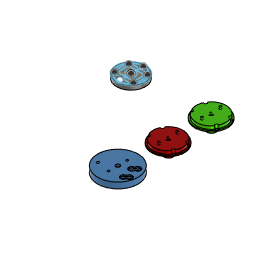
2023_05_26_IMacG4TopPart1 Fail v1 (Autodesk Fusion 360 design; units mm, degrees)
Autodesk Fusion 360 part; units mm, degrees
sketch "Screw Dim" plane through (0, 0, 0) normal (0, 0, 1) x (1, 0, 0)
  circle A0 centre (0, 0) radius 3.5
  circle A1 centre (0, 0) radius 1.755
  dimension "d1" = 7
  dimension "d2" = 3.51
  constraint coincident A0.centre A1.centre
  constraint concentric A0 A1
  measures "d1" diameter of A0
  measures "d2" diameter of A1
extrude "Extrude1" add sketch "Screw Dim" along normal blind 5 contours A0 | A1 makes body 1
extrude "Extrude2" cut sketch "Screw Dim" along normal blind 3.8 bodies 1
move_body "Move1" bodies 1 to x (1, 0, 0) y (0, 1, 0) z (0, 0, 1) at (0, 50, 0)
sketch "Sketch2" plane through (0, 0, 0) normal (0, 0, 1) x (1, 0, 0)
  line L0 (0, 0) -> (22.6, 0) construction
  line L1 (-10.9513, 2.215) -> (-10.9513, 17.585) construction
  line L2 (-10.9513, 9.9) -> (-10.9513, 22.015) construction
  line L3 (-10.9513, 9.9) -> (-10.9513, -2.215) construction
  line L4 (11.3, 0) -> (26.3, 0) construction
  line L5 (11.3, 0) -> (-3.7, 0) construction
  line L6 (-10.9513, 2.215) -> (-10.9513, -2.215) construction
  line L7 (-10.9513, 22.015) -> (-10.9513, 17.585) construction
  line L8 (26.3, 0) -> (22.6, 0) construction
  line L9 (-10.9513, 19.8) -> (24.45, 19.8) construction
  line L10 (24.45, 19.8) -> (24.45, 0) construction
  circle A0 centre (-10.9513, 19.8) radius 2.215
  circle A1 centre (24.45, 19.8) radius 2.215
  circle A2 centre (24.45, 0) radius 2.215
  circle A3 centre (-10.9513, 0) radius 2.215
  line L11 (-10.9513, 19.8) -> (24.45, 0) construction
  line L12 (24.45, 19.8) -> (-10.9513, 0) construction
  line L13 (6.7494, 9.9) -> (6.7494, 21.3) construction
  line L14 (6.7494, 9.9) -> (6.7494, 24.3) construction
  line L15 (6.7494, 21.3) -> (6.7494, 24.3) construction
  line L16 (6.7494, 9.9) -> (6.7494, -3.45) construction
  circle A4 centre (6.7494, 9.9) radius 2.875
  circle A5 centre (6.7494, 9.9) radius 11.35
  circle A6 centre (6.7494, 9.9) radius 20.6
  circle A7 centre (6.7494, 9.9) radius 22.6
  line L17 (0, 0) -> (-3.7, 0)
  circle A8 centre (6.7494, 22.8) radius 1.5
  circle A9 centre (6.7494, -3) radius 1.5
  line L18 (-10.9513, 22.015) -> (-10.9513, -2.215)
  point P0 (-10.9513, 0)
  point P1 (-10.9513, 0)
  point P2 (-1.85, 0)
  dimension "d10" = 22.6
  dimension "d11" = 15.37
  dimension "d12" = 12.115
  dimension "d13" = 12.115
  dimension "d14" = 15
  dimension "d15" = 14.4
  dimension "d16" = 11.4
  dimension "d18" = 5.75
  dimension "d19" = 41.2
  dimension "d20" = 45.2
  dimension "d56" = 360
  dimension "d66" = 24.23
  constraint coincident L0.start L17.start
  constraint horizontal L0
  constraint vertical L1
  constraint coincident L1 L2.start
  constraint parallel L1 L2
  constraint parallel L1 L3
  constraint midpoint L1 L2.start
  constraint midpoint L0 L4.start
  constraint parallel L0 L4
  constraint parallel L0 L5
  constraint equal L4 L5
  constraint coincident L5 P1
  constraint midpoint L6 P1
  constraint coincident P1 P0
  constraint midpoint L7 L9.start
  constraint perpendicular L7 L9
  constraint midpoint L8 L10.end
  constraint perpendicular L8 L10
  constraint coincident L9.start A0.centre
  constraint coincident L1.end A0
  constraint coincident L9.end L10.start
  constraint coincident L10.end A2.centre
  constraint equal A0 A1
  constraint equal A0 A3
  constraint equal A0 A2
  constraint midpoint L11 L13.start
  constraint perpendicular L9 L13
  constraint parallel L13 L14
  constraint parallel L14 L16
  constraint coincident L13.start L14.start
  constraint concentric A4 A5
  constraint concentric A4 A6
  constraint concentric A5 A7
  constraint midpoint L17 P2
  constraint coincident L14.end A8
  constraint coincident L13.end A8
  measures "d10" distance of L0.start L0.end
  measures "d11" distance of L1.start L1.end
  measures "d12" distance of L2.start L2.end
  measures "d13" distance of L2.start L3.end
  measures "d14" distance of L4.start L4.end
  measures "d15" distance of L13.start L14.end
  measures "d16" distance of L13.start L13.end
  measures "d18" diameter of A4
  measures "d19" diameter of A6
  measures "d20" diameter of A7
  measures "d66" distance of L2.end L3.end
extrude "Extrude3" add sketch "Sketch2" against normal blind 5.75 separate body contours A0 A6 L18 | A0 A1 A2 A3 A6 L18 | A0 A6 L18 | A0 A3 A6 L18 | A0 A6 L18 | A0 A6 L18 | A1 A6 | A1 A6 | A3 A6 L18 | A3 A6 L18 | A3 A6 L18 | A3 A6 L18 | A2 A6 | A2 A6 | A4 | A5 | A7 | A8 | A9 makes body 2
extrude "Extrude4" cut sketch "Sketch2" against normal blind 4.15 contours A0 A6 L18 | A0 A6 L18 | A1 A6 | A3 A6 L18 | A3 A6 L18 | A2 A6 | A7 picked at (-10.6589, 21.4307) picked at (-11.7417, 20.3274) picked at (25.2501, 20.2971) picked at (-11.7417, -0.5274) picked at (-10.6589, -1.6307) picked at (25.2501, -0.4971) bodies 2
extrude "Extrude5" cut sketch "Sketch2" against normal blind 5.2 contours A0 A6 L18 | A0 A6 L18 | A0 A6 L18 | A0 A6 L18 | A1 A6 | A1 A6 | A3 A6 L18 | A3 A6 L18 | A3 A6 L18 | A3 A6 L18 | A2 A6 | A2 A6 bodies 2
extrude "Extrude6" add sketch "Sketch2" along normal blind 2.5 contours A8 | A9 bodies 2
extrude "Extrude7" cut sketch "Sketch2" against normal blind 28 contours A4 bodies 2
sketch "Sketch10" plane through (0, 0, 0) normal (0, 0, 1) x (1, 0, 0)
  line L0 (-82.5, 14.73) -> (-112.5, 14.73)
  line L1 (-112.5, 14.73) -> (-112.5, -9.5)
  line L2 (-112.5, -9.5) -> (-82.5, -9.5)
  line L3 (-82.5, -9.5) -> (-82.5, 14.73)
  line L4 (-82.5, 14.73) -> (-112.5, -9.5) construction
  line L5 (-112.5, 14.73) -> (-82.5, -9.5) construction
  line L6 (-86.2, 10.3) -> (-108.8, 10.3)
  line L7 (-108.8, 10.3) -> (-108.8, -5.07)
  line L8 (-108.8, -5.07) -> (-86.2, -5.07)
  line L9 (-86.2, -5.07) -> (-86.2, 10.3)
  line L10 (-86.2, 10.3) -> (-108.8, -5.07) construction
  line L11 (-108.8, 10.3) -> (-86.2, -5.07) construction
  line L12 (-97.5, 2.615) -> (-97.5, 16.515)
  line L13 (-97.5, 2.615) -> (-97.5, 19.615)
  line L14 (-108.8, -5.07) -> (-112.5, -5.07) construction
  line L15 (-108.8, -5.07) -> (-108.8, -9.5) construction
  line L16 (-97.5, 19.615) -> (-97.5, -14.385)
  circle A0 centre (-97.5, 18.065) radius 1.55
  circle A1 centre (-97.5, -12.835) radius 1.55
  line L17 (-108.8, 10.3) -> (-112.5, 14.73) construction
  line L18 (-86.2, 10.3) -> (-82.5, 14.73) construction
  line L19 (-86.2, -5.07) -> (-82.5, -9.5) construction
  line L20 (-112.5, -9.5) -> (-108.8, -5.07) construction
  circle A2 centre (-110.65, 12.515) radius 1.7
  circle A3 centre (-84.35, 12.515) radius 1.7
  circle A4 centre (-84.35, -7.285) radius 1.7
  circle A5 centre (-110.65, -7.285) radius 1.7
  point P0 (-97.5, 2.615)
  point P1 (-97.5, 2.615)
  point P2 (-97.5, 19.615)
  dimension "d69" = 30
  dimension "d70" = 24.23
  dimension "d71" = 22.6
  dimension "d72" = 15.37
  dimension "d73" = 13.9
  dimension "d74" = 17
  dimension "d89" = 360
  dimension "d90" = 3.4
  constraint horizontal L0
  constraint perpendicular L0 L1
  constraint parallel L0 L2
  constraint parallel L1 L3
  constraint coincident L4 P1
  constraint coincident L5 P1
  constraint horizontal L6
  constraint perpendicular L6 L7
  constraint parallel L6 L8
  constraint parallel L7 L9
  constraint coincident L10 P1
  constraint coincident L11 P1
  constraint coincident P1 P0
  constraint perpendicular L0 L12
  constraint perpendicular L0 L13
  constraint coincident L1 L14.end
  constraint perpendicular L1 L14
  constraint coincident L2 L15.end
  constraint perpendicular L2 L15
  constraint perpendicular L2 L16
  constraint coincident P2 L13.end
  constraint coincident P2 A0
  constraint coincident L12.end A0
  constraint midpoint L17 A2.centre
  constraint midpoint L18 A3.centre
  constraint midpoint L19 A4.centre
  constraint midpoint L20 A5.centre
  constraint equal A2 A3
  constraint equal A2 A4
  constraint equal A2 A5
  measures "d69" distance of L1.end L2.end
  measures "d70" distance of L0.end L1.end
  measures "d71" distance of L7.end L8.end
  measures "d72" distance of L6.end L7.end
  measures "d73" distance of P1 L12.end
  measures "d74" distance of P1 P2
  measures "d90" diameter of A2
sketch "Sketch11" plane through (0, 0, 0) normal (0, 0, 1) x (1, 0, 0)
  line L0 (-113.85, -9.645) -> (-91.25, -9.645) construction
  line L1 (-91.25, -9.645) -> (-91.25, 5.725) construction
  line L2 (-91.25, 5.725) -> (-113.85, 5.725) construction
  line L3 (-113.85, 5.725) -> (-113.85, -9.645) construction
  line L4 (-108.8641, 10.1334) -> (-108.8641, -5.2366) construction
  line L5 (-108.8641, -5.2366) -> (-86.2641, -5.2366) construction
  line L6 (-86.2641, -5.2366) -> (-86.2641, 10.1334) construction
  line L7 (-86.2641, 10.1334) -> (-108.8641, 10.1334) construction
  line L8 (-108.8641, 10.1334) -> (-86.2641, -5.2366) construction
  line L9 (-108.8641, -5.2366) -> (-91.25, 5.725) construction
  circle A0 centre (-97.5641, 2.4484) radius 2.875
  circle A1 centre (-97.5641, 2.4484) radius 6
  circle A2 centre (-97.5641, 2.4484) radius 17.95
  circle A3 centre (-97.5641, 2.4484) radius 20
  dimension "d77" = 22.6
  dimension "d78" = 15.37
  dimension "d79" = 22.6
  dimension "d80" = 15.37
  dimension "d81" = 5.75
  dimension "d82" = 12
  dimension "d83" = 35.9
  dimension "d84" = 40
  constraint horizontal L2
  constraint perpendicular L2 L3
  constraint parallel L0 L2
  constraint parallel L1 L3
  constraint horizontal L7
  constraint perpendicular L4 L7
  constraint parallel L5 L7
  constraint parallel L4 L6
  constraint midpoint L8 A0.centre
  constraint concentric A0 A1
  constraint concentric A0 A2
  constraint concentric A2 A3
  measures "d77" distance of L0.end L0.start
  measures "d78" distance of L2.end L0.start
  measures "d79" distance of L5.end L4.end
  measures "d80" distance of L4.start L4.end
  measures "d81" diameter of A0
  measures "d82" diameter of A1
  measures "d83" diameter of A2
  measures "d84" diameter of A3
extrude "Extrude12" add sketch "Sketch11" against normal blind 5.7 separate body contours A1 | A2 | A3 makes body 3
sketch "Sketch3" plane through (0, 0, 0) normal (0, 0, 1) x (1, 0, 0)
  circle A0 centre (6.7494, 9.9) radius 5.35
  circle A1 centre (6.7494, 9.9) radius 6
  line L0 (-1.645, 7.9) -> (-1.645, -4.215) construction
  circle A2 centre (9.3, 7.9) radius 2.875
  point P0 (6.7494, 9.9)
  dimension "d31" = 10.7
  dimension "d32" = 12
  dimension "d57" = 12.115
  dimension "d58" = 5.75
  constraint concentric A0 A1
  constraint coincident P0 A0.centre
  measures "d31" diameter of A0
  measures "d32" diameter of A1
  measures "d57" distance of L0.end L0.start
  measures "d58" diameter of A2
sketch "Sketch4" plane through (0, 0, 0) normal (0, 0, 1) x (1, 0, 0)
sketch "Sketch5" plane through (0, 0, 0) normal (0, 0, 1) x (-1, 0, 0)
  circle A0 centre (-6.7494, -9.9) radius 20.6
  circle A1 centre (-6.7494, -9.9) radius 1.67
  circle A2 centre (-24.45, 0) radius 1.67
  circle A3 centre (10.9513, 0) radius 1.67
  circle A4 centre (-24.45, -19.8) radius 1.67
  circle A5 centre (-6.7494, -9.9) radius 28.0922
  circle A6 centre (-6.7494, 3) radius 1.5
  circle A7 centre (-6.7494, -22.8) radius 1.5
  circle A8 centre (-6.7494, -9.9) radius 2.875
  circle A9 centre (-6.7494, -9.9) radius 2.875
  arc A10 (10.0494, 2.0231) -> (12.203, -1.8274) centre (10.9513, 0) ccw
  arc A11 (10.0494, 2.0231) -> (-23.5482, 2.0231) centre (-6.7494, -9.9) ccw
  arc A12 (-25.7018, -1.8274) -> (-23.5482, 2.0231) centre (-24.45, 0) ccw
  arc A13 (-25.7018, -1.8274) -> (-25.7018, -17.9726) centre (-6.7494, -9.9) ccw
  arc A14 (-23.5482, -21.8231) -> (-25.7018, -17.9726) centre (-24.45, -19.8) ccw
  arc A15 (-23.5482, -21.8231) -> (10.0494, -21.8231) centre (-6.7494, -9.9) ccw
  arc A16 (12.203, -17.9726) -> (10.0494, -21.8231) centre (10.9513, -19.8) ccw
  arc A17 (12.203, -17.9726) -> (12.203, -1.8274) centre (-6.7494, -9.9) ccw
  constraint concentric A0 A5
  constraint coincident A0.centre A1.centre
  constraint coincident A3.centre A10.centre
  constraint coincident A4.centre A14.centre
  constraint coincident A2.centre A12.centre
extrude "Extrude10" add sketch "Sketch5" along normal blind 2.5 and the other way blind 5.75 separate body contours A0 A10 A11 A12 A13 A14 A15 A16 A17 | A0 A3 A10 | A0 A16 | A0 A2 A12 | A0 A4 A14 | A5 | A6 | A7 makes body 4
combine "Combine1" operation cut target body 4 tool bodies 2 keep tools
draft "Draft1" angle 24 neutral plane through (0, 50, 3.8) pull (0, 0, -1) 1 faces at (3.4826, 49.6515, 4.2) on bodies 1
copy_body "CopyPasteBodies1" bodies 1 makes body 5
move_body "Move2" bodies 5 to x (1, 0, 0) y (0, 1, 0) z (0, 0, 1) at (20.245, -34.2, -1.3)
copy_body "CopyPasteBodies2" bodies 5 makes body 6
move_body "Move3" bodies 6 to x (1, 0, 0) y (0, 1, 0) z (0, 0, 1) at (4.205, -15.8, 0)
copy_body "CopyPasteBodies3" bodies 5 6 makes body 7 makes body 8
move_body "Move4" bodies 7 8 to x (1, 0, 0) y (0, 1, 0) z (0, 0, 1) at (4.205, 4, 0)
move_body "Move5" bodies 7 8 6 5 to x (1, 0, 0) y (0, 1, 0) z (0, 0, 1) at (0, 0, -1.2)
combine "Combine2" operation cut target body 4 tool bodies 5 6 7 8 keep tools
move_body "Move6" bodies 7 8 6 5 to x (1, 0, 0) y (0, 1, 0) z (0, 0, 1) at (0, 0, 11)
fillet "Fillet1" radius 1.3 4 edges at (22.8138, 20.4346, 1.3) (18.6088, 16.4346, 1.3) (22.8138, 0.6346, 1.3) (27.0188, 4.6346, 1.3) on bodies 4
copy_body "CopyPasteBodies4" bodies 4 makes body 9
move_body "Move7" bodies 9 to x (1, 0, 0) y (0, 1, 0) z (0, 0, 1) at (0, -130, 0)
sketch "Sketch6" plane through (0, 0, 0) normal (0, 0, 1) x (-1, 0, 0)
  circle A0 centre (-6.7494, 3) radius 1.5
  circle A1 centre (-6.7494, -22.8) radius 1.5
  circle A2 centre (-6.7494, -9.9) radius 2.875
  arc A3 (10.0494, 2.0231) -> (12.203, -1.8274) centre (10.9513, 0) ccw
  arc A4 (10.0494, 2.0231) -> (-23.5482, 2.0231) centre (-6.7494, -9.9) ccw
  arc A5 (-25.7018, -1.8274) -> (-23.5482, 2.0231) centre (-24.45, 0) ccw
  arc A6 (-25.7018, -1.8274) -> (-25.7018, -17.9726) centre (-6.7494, -9.9) ccw
  arc A7 (-23.5482, -21.8231) -> (-25.7018, -17.9726) centre (-24.45, -19.8) ccw
  arc A8 (-23.5482, -21.8231) -> (10.0494, -21.8231) centre (-6.7494, -9.9) ccw
  arc A9 (12.203, -17.9726) -> (10.0494, -21.8231) centre (10.9513, -19.8) ccw
  arc A10 (12.203, -17.9726) -> (12.203, -1.8274) centre (-6.7494, -9.9) ccw
sketch "Sketch7" plane through (0, 0, 0) normal (0, 0, 1) x (1, 0, 0)
sketch "Sketch8" plane through (0, 0, 0) normal (0, 0, 1) x (-1, 0, 0)
  circle A0 centre (-9.3, -7.9) radius 20.6
  circle A1 centre (-9.3, -7.9) radius 2.875
  circle A2 centre (-9.3, -7.9) radius 6
  dimension "d62" = 5.75
  dimension "d63" = 12
  constraint concentric A0 A1
  constraint concentric A1 A2
  measures "d62" diameter of A1
  measures "d63" diameter of A2
extrude "Extrude11" add sketch "Sketch8" against normal blind 17 contours A2 bodies 2
sketch "TopImacG4Surface" plane through (0, 0, 0) normal (0, 0, 1) x (-1, 0, 0)
  circle A0 centre (-9.3, -7.9) radius 20.6
  circle A1 centre (-20.245, -15.8) radius 1.67
  circle A2 centre (-20.245, 0) radius 1.67
  circle A3 centre (1.645, 0) radius 1.67
  circle A4 centre (1.645, -15.8) radius 1.67
  circle A5 centre (-9.3, -20.8) radius 1.5
  circle A6 centre (-9.3, 5) radius 1.5
copy_body "CopyPasteBodies5" bodies 2 makes body 10
move_body "Move8" bodies 10 to x (1, 0, 0) y (0, 1, 0) z (0, 0, 1) at (0, -60, 0)
hidden bodies 4
equation "d5 = 5 mm - 1.2 mm"
equation "d10 = xmin"
equation "d11 = ymin"
equation "d12 = ymax / 2"
equation "d13 = d12"
equation "d14 = xmax / 2"
equation "d15 = ( 28.8 / 2 ) * 1 mm"
equation "d16 = ( 22.8 / 2 ) * 1 mm"
equation "d23 = -5.75 mm + 1.6 mm"
equation "xmax = 30 mm"
equation "xmin = 22.6 mm"
equation "ymax = 24.23 mm"
equation "ymin = 15.37 mm"
equation "d57 = d12"
equation "middlemin = 27.8 mm"
equation "middlemax = 34 mm"
equation "d69 = xmax"
equation "d70 = ymax"
equation "d71 = xmin"
equation "d72 = ymin"
equation "d73 = middlemin / 2"
equation "d74 = middlemax / 2"
equation "d77 = xmin"
equation "d78 = ymin"
equation "d79 = xmin"
equation "d80 = ymin"
equation "d83 = ( 35.9 / 1 ) * 1 mm"
equation "d84 = ( 40 / 1 ) * 1 mm"
named bodies: "Screw", "Top Part Imac G4", "ToPartImacG4 Wrapper", "Screw (1)", "Screw (1) (1)", "Screw (1) (1) (1)", "Screw (1) (1) (1) (1)", "ToPartImacG4 Wrapper (1)", "Top Part Imac G4 (1)"
